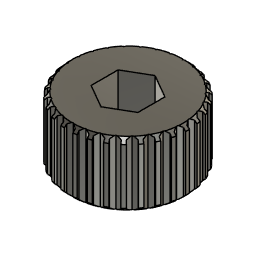
Knob v7 (Autodesk Fusion 360 design; units mm, degrees)
Autodesk Fusion 360 part; units mm, degrees
sketch "Sketch1" plane through (0, 0, 0) normal (0, 0, 1) x (1, 0, 0) in component "Component"
  circle A0 centre (0, 0) radius 14
  circle A1 centre (0, 0) radius 3.5
  line L0 (5.5, 3.1754) -> (0, 6.3509)
  line L1 (0, 6.3509) -> (-5.5, 3.1754)
  line L2 (-5.5, 3.1754) -> (-5.5, -3.1754)
  line L3 (-5.5, -3.1754) -> (0, -6.3509)
  line L4 (0, -6.3509) -> (5.5, -3.1754)
  line L5 (5.5, -3.1754) -> (5.5, 3.1754)
  line L6 (0, 0) -> (0, -14) construction
  line L7 (0, -14) -> (5, -14) construction
  line L8 (1, -13.4226) -> (0, -12.8453)
  line L9 (0, -12.8453) -> (-1, -13.4226)
  line L10 (-1, -13.4226) -> (-1, -14.5774)
  line L11 (-1, -14.5774) -> (0, -15.1547)
  line L12 (0, -15.1547) -> (1, -14.5774)
  line L13 (1, -14.5774) -> (1, -13.4226)
  line L14 (3.1508, -14.8235) -> (4.0089, -14.0509)
  line L15 (3.7689, -12.9214) -> (2.6707, -12.5646)
  line L16 (4.0089, -14.0509) -> (3.7689, -12.9214)
  line L17 (2.0527, -14.4667) -> (3.1508, -14.8235)
  line L18 (1.8126, -13.3372) -> (2.0527, -14.4667)
  line L19 (2.6707, -12.5646) -> (1.8126, -13.3372)
  line L20 (6.164, -13.8445) -> (6.8427, -12.9103)
  line L21 (6.373, -11.8555) -> (5.2247, -11.7348)
  line L22 (6.8427, -12.9103) -> (6.373, -11.8555)
  line L23 (5.0156, -13.7238) -> (6.164, -13.8445)
  line L24 (4.5459, -12.6689) -> (5.0156, -13.7238)
  line L25 (5.2247, -11.7348) -> (4.5459, -12.6689)
  line L26 (8.9077, -12.2604) -> (9.3774, -11.2055)
  line L27 (8.6987, -10.2714) -> (7.5503, -10.3921)
  line L28 (9.3774, -11.2055) -> (8.6987, -10.2714)
  line L29 (7.7593, -12.3811) -> (8.9077, -12.2604)
  line L30 (7.0806, -11.4469) -> (7.7593, -12.3811)
  line L31 (7.5503, -10.3921) -> (7.0806, -11.4469)
  line L32 (11.2621, -10.1405) -> (11.5022, -9.011)
  line L33 (10.6441, -8.2384) -> (9.5459, -8.5952)
  line L34 (11.5022, -9.011) -> (10.6441, -8.2384)
  line L35 (10.164, -10.4973) -> (11.2621, -10.1405)
  line L36 (9.3058, -9.7247) -> (10.164, -10.4973)
  line L37 (9.5459, -8.5952) -> (9.3058, -9.7247)
  line L38 (13.1244, -7.5774) -> (13.1244, -6.4226)
  line L39 (12.1244, -5.8453) -> (11.1244, -6.4226)
  line L40 (13.1244, -6.4226) -> (12.1244, -5.8453)
  line L41 (12.1244, -8.1547) -> (13.1244, -7.5774)
  line L42 (11.1244, -7.5774) -> (12.1244, -8.1547)
  line L43 (11.1244, -6.4226) -> (11.1244, -7.5774)
  line L44 (14.413, -4.6831) -> (14.1729, -3.5536)
  line L45 (13.0747, -3.1968) -> (12.2166, -3.9694)
  line L46 (14.1729, -3.5536) -> (13.0747, -3.1968)
  line L47 (13.5549, -5.4557) -> (14.413, -4.6831)
  line L48 (12.4567, -5.0989) -> (13.5549, -5.4557)
  line L49 (12.2166, -3.9694) -> (12.4567, -5.0989)
  line L50 (15.0717, -1.5841) -> (14.602, -0.5292)
  line L51 (13.4536, -0.4085) -> (12.7749, -1.3427)
  line L52 (14.602, -0.5292) -> (13.4536, -0.4085)
  line L53 (14.393, -2.5183) -> (15.0717, -1.5841)
  line L54 (13.2446, -2.3976) -> (14.393, -2.5183)
  line L55 (12.7749, -1.3427) -> (13.2446, -2.3976)
  line L56 (15.0717, 1.5841) -> (14.393, 2.5183)
  line L57 (13.2446, 2.3976) -> (12.7749, 1.3427)
  line L58 (14.393, 2.5183) -> (13.2446, 2.3976)
  line L59 (14.602, 0.5292) -> (15.0717, 1.5841)
  line L60 (13.4536, 0.4085) -> (14.602, 0.5292)
  line L61 (12.7749, 1.3427) -> (13.4536, 0.4085)
  line L62 (14.413, 4.6831) -> (13.5549, 5.4557)
  line L63 (12.4567, 5.0989) -> (12.2166, 3.9694)
  line L64 (13.5549, 5.4557) -> (12.4567, 5.0989)
  line L65 (14.1729, 3.5536) -> (14.413, 4.6831)
  line L66 (13.0747, 3.1968) -> (14.1729, 3.5536)
  line L67 (12.2166, 3.9694) -> (13.0747, 3.1968)
  line L68 (13.1244, 7.5774) -> (12.1244, 8.1547)
  line L69 (11.1244, 7.5774) -> (11.1244, 6.4226)
  line L70 (12.1244, 8.1547) -> (11.1244, 7.5774)
  line L71 (13.1244, 6.4226) -> (13.1244, 7.5774)
  line L72 (12.1244, 5.8453) -> (13.1244, 6.4226)
  line L73 (11.1244, 6.4226) -> (12.1244, 5.8453)
  line L74 (11.2621, 10.1405) -> (10.164, 10.4973)
  line L75 (9.3058, 9.7247) -> (9.5459, 8.5952)
  line L76 (10.164, 10.4973) -> (9.3058, 9.7247)
  line L77 (11.5022, 9.011) -> (11.2621, 10.1405)
  line L78 (10.6441, 8.2384) -> (11.5022, 9.011)
  line L79 (9.5459, 8.5952) -> (10.6441, 8.2384)
  line L80 (8.9077, 12.2604) -> (7.7593, 12.3811)
  line L81 (7.0806, 11.4469) -> (7.5503, 10.3921)
  line L82 (7.7593, 12.3811) -> (7.0806, 11.4469)
  line L83 (9.3774, 11.2055) -> (8.9077, 12.2604)
  line L84 (8.6987, 10.2714) -> (9.3774, 11.2055)
  line L85 (7.5503, 10.3921) -> (8.6987, 10.2714)
  line L86 (6.164, 13.8445) -> (5.0156, 13.7238)
  line L87 (4.5459, 12.6689) -> (5.2247, 11.7348)
  line L88 (5.0156, 13.7238) -> (4.5459, 12.6689)
  line L89 (6.8427, 12.9103) -> (6.164, 13.8445)
  line L90 (6.373, 11.8555) -> (6.8427, 12.9103)
  line L91 (5.2247, 11.7348) -> (6.373, 11.8555)
  line L92 (3.1508, 14.8235) -> (2.0527, 14.4667)
  line L93 (1.8126, 13.3372) -> (2.6707, 12.5646)
  line L94 (2.0527, 14.4667) -> (1.8126, 13.3372)
  line L95 (4.0089, 14.0509) -> (3.1508, 14.8235)
  line L96 (3.7689, 12.9214) -> (4.0089, 14.0509)
  line L97 (2.6707, 12.5646) -> (3.7689, 12.9214)
  line L98 (0, 15.1547) -> (-1, 14.5774)
  line L99 (-1, 13.4226) -> (0, 12.8453)
  line L100 (-1, 14.5774) -> (-1, 13.4226)
  line L101 (1, 14.5774) -> (0, 15.1547)
  line L102 (1, 13.4226) -> (1, 14.5774)
  line L103 (0, 12.8453) -> (1, 13.4226)
  line L104 (-3.1508, 14.8235) -> (-4.0089, 14.0509)
  line L105 (-3.7689, 12.9214) -> (-2.6707, 12.5646)
  line L106 (-4.0089, 14.0509) -> (-3.7689, 12.9214)
  line L107 (-2.0527, 14.4667) -> (-3.1508, 14.8235)
  line L108 (-1.8126, 13.3372) -> (-2.0527, 14.4667)
  line L109 (-2.6707, 12.5646) -> (-1.8126, 13.3372)
  line L110 (-6.164, 13.8445) -> (-6.8427, 12.9103)
  line L111 (-6.373, 11.8555) -> (-5.2247, 11.7348)
  line L112 (-6.8427, 12.9103) -> (-6.373, 11.8555)
  line L113 (-5.0156, 13.7238) -> (-6.164, 13.8445)
  line L114 (-4.5459, 12.6689) -> (-5.0156, 13.7238)
  line L115 (-5.2247, 11.7348) -> (-4.5459, 12.6689)
  line L116 (-8.9077, 12.2604) -> (-9.3774, 11.2055)
  line L117 (-8.6987, 10.2714) -> (-7.5503, 10.3921)
  line L118 (-9.3774, 11.2055) -> (-8.6987, 10.2714)
  line L119 (-7.7593, 12.3811) -> (-8.9077, 12.2604)
  line L120 (-7.0806, 11.4469) -> (-7.7593, 12.3811)
  line L121 (-7.5503, 10.3921) -> (-7.0806, 11.4469)
  line L122 (-11.2621, 10.1405) -> (-11.5022, 9.011)
  line L123 (-10.6441, 8.2384) -> (-9.5459, 8.5952)
  line L124 (-11.5022, 9.011) -> (-10.6441, 8.2384)
  line L125 (-10.164, 10.4973) -> (-11.2621, 10.1405)
  line L126 (-9.3058, 9.7247) -> (-10.164, 10.4973)
  line L127 (-9.5459, 8.5952) -> (-9.3058, 9.7247)
  line L128 (-13.1244, 7.5774) -> (-13.1244, 6.4226)
  line L129 (-12.1244, 5.8453) -> (-11.1244, 6.4226)
  line L130 (-13.1244, 6.4226) -> (-12.1244, 5.8453)
  line L131 (-12.1244, 8.1547) -> (-13.1244, 7.5774)
  line L132 (-11.1244, 7.5774) -> (-12.1244, 8.1547)
  line L133 (-11.1244, 6.4226) -> (-11.1244, 7.5774)
  line L134 (-14.413, 4.6831) -> (-14.1729, 3.5536)
  line L135 (-13.0747, 3.1968) -> (-12.2166, 3.9694)
  line L136 (-14.1729, 3.5536) -> (-13.0747, 3.1968)
  line L137 (-13.5549, 5.4557) -> (-14.413, 4.6831)
  line L138 (-12.4567, 5.0989) -> (-13.5549, 5.4557)
  line L139 (-12.2166, 3.9694) -> (-12.4567, 5.0989)
  line L140 (-15.0717, 1.5841) -> (-14.602, 0.5292)
  line L141 (-13.4536, 0.4085) -> (-12.7749, 1.3427)
  line L142 (-14.602, 0.5292) -> (-13.4536, 0.4085)
  line L143 (-14.393, 2.5183) -> (-15.0717, 1.5841)
  line L144 (-13.2446, 2.3976) -> (-14.393, 2.5183)
  line L145 (-12.7749, 1.3427) -> (-13.2446, 2.3976)
  line L146 (-15.0717, -1.5841) -> (-14.393, -2.5183)
  line L147 (-13.2446, -2.3976) -> (-12.7749, -1.3427)
  line L148 (-14.393, -2.5183) -> (-13.2446, -2.3976)
  line L149 (-14.602, -0.5292) -> (-15.0717, -1.5841)
  line L150 (-13.4536, -0.4085) -> (-14.602, -0.5292)
  line L151 (-12.7749, -1.3427) -> (-13.4536, -0.4085)
  line L152 (-14.413, -4.6831) -> (-13.5549, -5.4557)
  line L153 (-12.4567, -5.0989) -> (-12.2166, -3.9694)
  line L154 (-13.5549, -5.4557) -> (-12.4567, -5.0989)
  line L155 (-14.1729, -3.5536) -> (-14.413, -4.6831)
  line L156 (-13.0747, -3.1968) -> (-14.1729, -3.5536)
  line L157 (-12.2166, -3.9694) -> (-13.0747, -3.1968)
  line L158 (-13.1244, -7.5774) -> (-12.1244, -8.1547)
  line L159 (-11.1244, -7.5774) -> (-11.1244, -6.4226)
  line L160 (-12.1244, -8.1547) -> (-11.1244, -7.5774)
  line L161 (-13.1244, -6.4226) -> (-13.1244, -7.5774)
  line L162 (-12.1244, -5.8453) -> (-13.1244, -6.4226)
  line L163 (-11.1244, -6.4226) -> (-12.1244, -5.8453)
  line L164 (-11.2621, -10.1405) -> (-10.164, -10.4973)
  line L165 (-9.3058, -9.7247) -> (-9.5459, -8.5952)
  line L166 (-10.164, -10.4973) -> (-9.3058, -9.7247)
  line L167 (-11.5022, -9.011) -> (-11.2621, -10.1405)
  line L168 (-10.6441, -8.2384) -> (-11.5022, -9.011)
  line L169 (-9.5459, -8.5952) -> (-10.6441, -8.2384)
  line L170 (-8.9077, -12.2604) -> (-7.7593, -12.3811)
  line L171 (-7.0806, -11.4469) -> (-7.5503, -10.3921)
  line L172 (-7.7593, -12.3811) -> (-7.0806, -11.4469)
  line L173 (-9.3774, -11.2055) -> (-8.9077, -12.2604)
  line L174 (-8.6987, -10.2714) -> (-9.3774, -11.2055)
  line L175 (-7.5503, -10.3921) -> (-8.6987, -10.2714)
  line L176 (-6.164, -13.8445) -> (-5.0156, -13.7238)
  line L177 (-4.5459, -12.6689) -> (-5.2247, -11.7348)
  line L178 (-5.0156, -13.7238) -> (-4.5459, -12.6689)
  line L179 (-6.8427, -12.9103) -> (-6.164, -13.8445)
  line L180 (-6.373, -11.8555) -> (-6.8427, -12.9103)
  line L181 (-5.2247, -11.7348) -> (-6.373, -11.8555)
  line L182 (-3.1508, -14.8235) -> (-2.0527, -14.4667)
  line L183 (-1.8126, -13.3372) -> (-2.6707, -12.5646)
  line L184 (-2.0527, -14.4667) -> (-1.8126, -13.3372)
  line L185 (-4.0089, -14.0509) -> (-3.1508, -14.8235)
  line L186 (-3.7689, -12.9214) -> (-4.0089, -14.0509)
  line L187 (-2.6707, -12.5646) -> (-3.7689, -12.9214)
  point P0 (0, -14)
  point P1 (2.9108, -13.6941)
  point P2 (2.9108, -13.6941)
  point P3 (5.6943, -12.7896)
  point P4 (5.6943, -12.7896)
  point P5 (8.229, -11.3262)
  point P6 (8.229, -11.3262)
  point P7 (10.404, -9.3678)
  point P8 (10.404, -9.3678)
  point P9 (12.1244, -7)
  point P10 (12.1244, -7)
  point P11 (13.3148, -4.3262)
  point P12 (13.3148, -4.3262)
  point P13 (13.9233, -1.4634)
  point P14 (13.9233, -1.4634)
  point P15 (13.9233, 1.4634)
  point P16 (13.9233, 1.4634)
  point P17 (13.3148, 4.3262)
  point P18 (13.3148, 4.3262)
  point P19 (12.1244, 7)
  point P20 (12.1244, 7)
  point P21 (10.404, 9.3678)
  point P22 (10.404, 9.3678)
  point P23 (8.229, 11.3262)
  point P24 (8.229, 11.3262)
  point P25 (5.6943, 12.7896)
  point P26 (5.6943, 12.7896)
  point P27 (2.9108, 13.6941)
  point P28 (2.9108, 13.6941)
  point P29 (0, 14)
  point P30 (0, 14)
  point P31 (-2.9108, 13.6941)
  point P32 (-2.9108, 13.6941)
  point P33 (-5.6943, 12.7896)
  point P34 (-5.6943, 12.7896)
  point P35 (-8.229, 11.3262)
  point P36 (-8.229, 11.3262)
  point P37 (-10.404, 9.3678)
  point P38 (-10.404, 9.3678)
  point P39 (-12.1244, 7)
  point P40 (-12.1244, 7)
  point P41 (-13.3148, 4.3262)
  point P42 (-13.3148, 4.3262)
  point P43 (-13.9233, 1.4634)
  point P44 (-13.9233, 1.4634)
  point P45 (-13.9233, -1.4634)
  point P46 (-13.9233, -1.4634)
  point P47 (-13.3148, -4.3262)
  point P48 (-13.3148, -4.3262)
  point P49 (-12.1244, -7)
  point P50 (-12.1244, -7)
  point P51 (-10.404, -9.3678)
  point P52 (-10.404, -9.3678)
  point P53 (-8.229, -11.3262)
  point P54 (-8.229, -11.3262)
  point P55 (-5.6943, -12.7896)
  point P56 (-5.6943, -12.7896)
  point P57 (-2.9108, -13.6941)
  point P58 (-2.9108, -13.6941)
  dimension "d1" = 28
  dimension "d2" = 7
  dimension "d3" = 5.5
  dimension "d16" = 5
  dimension "d17" = 1
  dimension "d19" = 360
  constraint coincident A0.centre A1.centre
  constraint concentric A0 A1
  constraint coincident A0 P0
  constraint parallel L5 L6
  constraint tangent A0 L7
  constraint coincident P0 L6.end
  measures "d1" diameter of A0
  measures "d2" diameter of A1
  measures "d3" distance of A0.centre L5
  measures "d16" distance of P0 L7.end
  measures "d17" distance of P0 L13
extrude "Extrude1" add sketch "Sketch1" along normal blind 8 contours A0 L8 L9 L10 L13 L15 L16 L18 L19 L21 L22 L24 L25 L27 L28 L30 L31 L33 L34 L36 L37 L39 L40 L42 L43 L45 L46 L48 L49 L51 L52 L54 L55 L57 L58 L60 L61 L63 L64 L66 L67 L69 L70 L72 L73 L75 L76 L78 L79 L81 L82 L84 L85 L87 L88 L90 L91 L93 L94 L96 L97 L99 L100 L102 L103 L105 L106 L108 L109 L111 L112 L114 L115 L117 L118 L120 L121 L123 L124 L126 L127 L129 L130 L132 L133 L135 L136 L138 L139 L141 L142 L144 L145 L147 L148 L150 L151 L153 L154 L156 L157 L159 L160 L162 L163 L165 L166 L168 L169 L171 L172 L174 L175 L177 L178 L180 L181 L183 L184 L186 L187 | A0 L57 L58 L60 L61 | A0 L51 L52 L54 L55 | A0 L63 L64 L66 L67 | A0 L45 L46 L48 L49 | A0 L69 L70 L72 L73 | A0 L39 L40 L42 L43 | A0 L75 L76 L78 L79 | A0 L33 L34 L36 L37 | A0 L81 L82 L84 L85 | A0 L27 L28 L30 L31 | A0 L87 L88 L90 L91 | A0 L21 L22 L24 L25 | A0 L93 L94 L96 L97 | A0 L15 L16 L18 L19 | A0 L99 L100 L102 L103 | A0 L8 L9 L10 L13 | A0 L105 L106 L108 L109 | A0 L183 L184 L186 L187 | A0 L111 L112 L114 L115 | A0 L177 L178 L180 L181 | A0 L117 L118 L120 L121 | A0 L171 L172 L174 L175 | A0 L123 L124 L126 L127 | A0 L165 L166 L168 L169 | A0 L129 L130 L132 L133 | A0 L159 L160 L162 L163 | A0 L135 L136 L138 L139 | A0 L153 L154 L156 L157 | A0 L141 L142 L144 L145 | A0 L147 L148 L150 L151 | L0 L1 L2 L3 L4 L5 in component "Component"
extrude "Extrude2" cut sketch "Sketch1" against normal blind 4.7 from surface at 8 contours L0 L1 L2 L3 L4 L5 in component "Component"
extrude "Extrude5" add 1 faces at (8.3333, 0, 8) along direction (0, 0, 1) blind 7 in component "Component"
chamfer "Chamfer1" distance 1 angle 45 2 edges at (-13.0526, -5.0626, 0) (-13.0526, -5.0626, 15) in component "Component"
extrude "Extrude4" cut sketch "Sketch1" along normal up to surface (15 mm away) contours A0 L57 L58 L60 L61 | A0 L56 L58 L59 L60 | A0 L50 L52 L53 L54 | A0 L51 L52 L54 L55 | A0 L63 L64 L66 L67 | A0 L62 L64 L65 L66 | A0 L44 L46 L47 L48 | A0 L45 L46 L48 L49 | A0 L69 L70 L72 L73 | A0 L68 L70 L71 L72 | A0 L38 L40 L41 L42 | A0 L39 L40 L42 L43 | A0 L75 L76 L78 L79 | A0 L74 L76 L77 L78 | A0 L32 L34 L35 L36 | A0 L33 L34 L36 L37 | A0 L81 L82 L84 L85 | A0 L80 L82 L83 L84 | A0 L26 L28 L29 L30 | A0 L27 L28 L30 L31 | A0 L87 L88 L90 L91 | A0 L86 L88 L89 L90 | A0 L20 L22 L23 L24 | A0 L21 L22 L24 L25 | A0 L93 L94 L96 L97 | A0 L92 L94 L95 L96 | A0 L14 L16 L17 L18 | A0 L15 L16 L18 L19 | A0 L99 L100 L102 L103 | A0 L98 L100 L101 L102 | A0 L10 L11 L12 L13 | A0 L8 L9 L10 L13 | A0 L105 L106 L108 L109 | A0 L104 L106 L107 L108 | A0 L182 L184 L185 L186 | A0 L183 L184 L186 L187 | A0 L111 L112 L114 L115 | A0 L110 L112 L113 L114 | A0 L176 L178 L179 L180 | A0 L177 L178 L180 L181 | A0 L117 L118 L120 L121 | A0 L116 L118 L119 L120 | A0 L170 L172 L173 L174 | A0 L171 L172 L174 L175 | A0 L123 L124 L126 L127 | A0 L122 L124 L125 L126 | A0 L164 L166 L167 L168 | A0 L165 L166 L168 L169 | A0 L129 L130 L132 L133 | A0 L128 L130 L131 L132 | A0 L158 L160 L161 L162 | A0 L159 L160 L162 L163 | A0 L135 L136 L138 L139 | A0 L134 L136 L137 L138 | A0 L152 L154 L155 L156 | A0 L153 L154 L156 L157 | A0 L141 L142 L144 L145 | A0 L140 L142 L143 L144 | A0 L146 L148 L149 L150 | A0 L147 L148 L150 L151 in component "Component"
component "Component" placed x (1, 0, 0) y (0, 1, 0) z (0, 0, 1) at (0, 0, 0)
equation "d3 = ( 11 / 2 ) * 1 mm"
